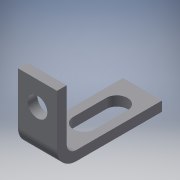
# Autodesk Inventor part: dsub37Bracket
Saved by Autodesk Inventor 2017 (Build 210142000, 142)
## iProperties
Created: 2016-10-03
Part Number: dsub37Bracket
Material: Generic
Document SubType Name: Sheet Metal
Designer: Zara
Density: 1 g/cm^3
Sheet Metal Rule: Default
Appearance: Default
Author: Zara
Autodesk Inventor part; units mm, degrees
ref_plane "YZ Plane" through (0, 0, 0) normal (1, 0, 0) x (0, 1, 0)
ref_plane "XZ Plane" through (0, 0, 0) normal (0, 1, 0) x (-1, 0, 0)
ref_plane "XY Plane" through (0, 0, 0) normal (0, 0, 1) x (1, 0, 0)
sketch "Sketch1" plane through (0, 0, 0) normal (0, 1, 0) x (-1, 0, 0)
  line L0 (-3.0226, 8.128) -> (3.0226, 8.128)
  line L1 (3.0226, 8.128) -> (3.0226, -8.128)
  line L2 (3.0226, -8.128) -> (-3.0226, -8.128)
  line L3 (-3.0226, -8.128) -> (-3.0226, 8.128)
  line L4 (-3.0226, 8.128) -> (3.0226, -8.128) construction
  line L5 (3.0226, 8.128) -> (-3.0226, -8.128) construction
  line L6 (1.651, 0.9398) -> (1.651, -4.3454)
  line L7 (-1.651, 0.9398) -> (-1.651, -4.3454)
  arc A0 (-1.651, -4.3454) -> (1.651, -4.3454) centre (0, -4.1402) ccw
  arc A1 (1.651, 0.9398) -> (-1.651, 0.9398) centre (0, 0.9398) ccw
  line L8 (0, 9.1418) -> (0, -10.0518)
  point P0 (0, 0)
  point P1 (0, 8.128)
  dimension "d0" = 16.256
  dimension "d1" = 6.0452
  dimension "d27" = 3.302
  dimension "d28" = 1.6637
  dimension "d29" = 3.0226
  dimension "d30" = 5.08
  measures "d0" distance of L0.end L1.end
  measures "d1" distance of L1.end L2.end
  measures "d27" distance between parallel lines of L7 L6
  measures "d28" radius of A0
  measures "d29" distance from line of A0.centre L1
  measures "d30" distance of A1.centre A0.centre
extrude "Plate1" add sketch "Sketch1" along normal blind 1.4986 contours L0 L8 A1 L7 A0 L2 L3 | L0 L1 L2 L8 A0 L6 A1
sketch "Sketch2" plane through (3.0226, 0, 6.6294) normal (0, 0, 1) x (1, 0, 0)
  line L0 (-6.0452, 0) -> (0, 0)
  line L1 (0, 0) -> (0, 10.922)
  line L2 (0, 10.922) -> (-6.0452, 10.922)
  line L3 (-6.0452, 10.922) -> (-6.0452, 0)
  constraints: 6 end point, 1 horizontal, 1 perpendicular, 1 vertical
edge flange "Flange1" height 10.922 angle 90 thickness 1.4986 bend radius 1.4986 thickness toward (0, 0, 1) relief straight relief width 1.4986 relief depth 0.7493 edges at (0, 1.4986, 8.128) wall of the first edge with corners at (-3.0226, 0, 6.6294) (3.0226, 0, 6.6294) (3.0226, 10.922, 6.6294) (-3.0226, 10.922, 6.6294)
bend "Bend1"
corner "Corner1"
sketch "Sketch4" plane through (3.0226, 10.922, 6.6294) normal (0, 0, -1) x (-1, 0, 0)
  circle A0 centre (3.0226, -3.683) radius 1.524
  line L0 (6.0452, 0) -> (0, 0) projected
  line L1 (0, -10.922) -> (6.0452, -10.922) projected
  point P0 (3.0226, -10.922)
  dimension "d22" = 3.048
  dimension "d25" = 7.239
  constraints: 1 centre point
  measures "d22" diameter of A0
  measures "d25" distance from line of L1 A0.centre
extrude "Extrusion3" cut sketch "Sketch4" against normal blind 1.4986
equation "\"d11\" = BendReliefWidth"
equation "\"d12\" = BendReliefDepth"
equation "\"d13\" = MinimumRemnant"
equation "\"d14\" = BendRadius"
equation "\"d17\" = BendRadius"
equation "\"d18\" = CornerReliefSize"
equation "\"d19\" = GapSize"
equation "\"d20\" = JacobiRadiusSize"
equation "\"BendRadius\" = Thickness"
equation "\"BendReliefWidth\" = Thickness"
equation "\"BendReliefDepth\" = 0.5 * Thickness"
equation "\"CornerReliefSize\" = 4 * Thickness"
equation "\"MinimumRemnant\" = 2 * Thickness"
equation "\"TransitionRadius\" = BendRadius"
equation "\"JacobiRadiusSize\" = Thickness"
equation "\"GapSize\" = Thickness"
equation "\"d10\" = BendRadius"
equation "\"Thickness\" = 1.4986"
body "Solid3"
